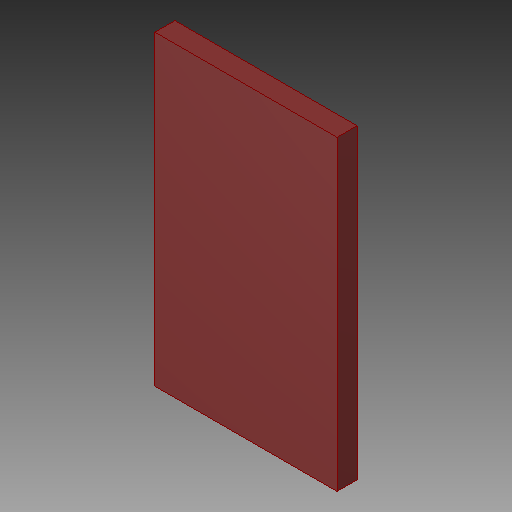
# Autodesk Inventor part: J5_2X3-SHROUDED
Saved by Autodesk Inventor 2017 (Build 210142000, 142)
## iProperties
Created: 2019-06-13
Part Number: J5_2X3-SHROUDED
Material: Generic
Document SubType Name: Modeling
Designer: Marc
Density: 1 g/cm^3
Appearance: 2X3-SHROUDED, J5_2X3-SHROUDED
Author: Marc
Autodesk Inventor part; units mm, degrees
ref_plane "YZ Plane" through (0, 0, 0) normal (1, 0, 0) x (0, 1, 0)
ref_plane "XZ Plane" through (0, 0, 0) normal (0, 1, 0) x (-1, 0, 0)
ref_plane "XY Plane" through (0, 0, 0) normal (0, 0, 1) x (1, 0, 0)
sketch "2X3-SHROUDED, J5_2X3-SHROUDED_58" plane through (0, 0, 0) normal (0, 0, 1) x (1, 0, 0)
  line L0 (-4.5, 7.6616) -> (4.6016, 7.6616)
  line L1 (4.6016, 7.6616) -> (4.6016, -7.6616)
  line L2 (4.6016, -7.6616) -> (-4.5, -7.6616)
  line L3 (-4.5, -7.6616) -> (-4.5, 7.6616)
  constraints: 8 end point
extrude "Extrusion1" add sketch "2X3-SHROUDED, J5_2X3-SHROUDED_58" along normal blind 1
body "Solid1"
